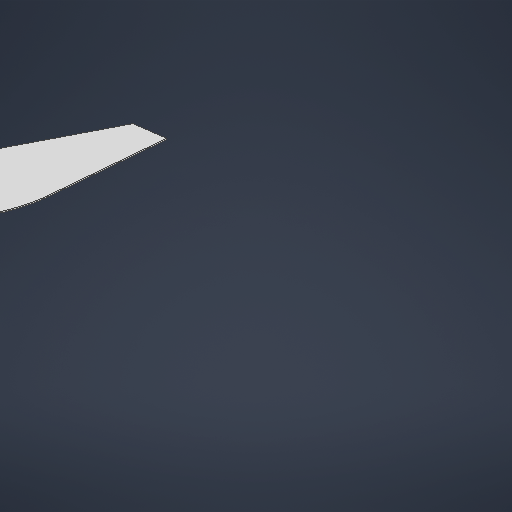
# Autodesk Inventor part: SLING
Saved by Autodesk Inventor 2026.2 (Build 302298010, 298A)
## iProperties
Created: 2026-04-04
Part Number: SLING
Material: Generic
Document SubType Name: Sheet Metal
Designer: 4aida
Density: 1 g/cm^3
Sheet Metal Rule: Default_mm
Appearance: Default
Author: 4aida
Autodesk Inventor part; units mm, degrees
ref_plane "YZ Plane" through (0, 0, 0) normal (1, 0, 0) x (0, 1, 0)
ref_plane "XZ Plane" through (0, 0, 0) normal (0, 1, 0) x (-1, 0, 0)
ref_plane "XY Plane" through (0, 0, 0) normal (0, 0, 1) x (1, 0, 0)
sketch "Sketch1" plane through (0, 0, 0) normal (0, 1, 0) x (-1, 0, 0)
  ellipse E0 centre (0, 0) end of major axis (0, -40) minor radius 25
  line L0 (23.4617, 13.8144) -> (8.75, 77.7778)
  line L1 (8.75, 77.7778) -> (-8.75, 77.7778)
  line L2 (-8.75, 77.7778) -> (-23.4617, 13.8144)
  line L3 (23.4617, -13.8144) -> (8.75, -77.7778)
  line L4 (8.75, -77.7778) -> (-8.75, -77.7778)
  line L5 (-8.75, -77.7778) -> (-23.4617, -13.8144)
  point P0 (0, 77.7778)
  point P1 (0, -77.7778)
  dimension "d0" = 25
  dimension "d1" = 40
  dimension "d2" = 77.7778
  dimension "d3" = 77.7778
  dimension "d5" = 17.5
  dimension "d7" = 17.5
  measures "d2" distance from line of point (0, 0) L1
  measures "d3" distance from line of L4 point (0, 0)
  measures "d5" distance of L0.end L1.end
  measures "d7" distance of L3.end L4.end
extrude "Plate1" add sketch "Sketch1" along normal blind 0.5
equation "\"d2\" = d3"
equation "\"d3\" = 3.11111 * d0"
equation "\"d5\" = d7"
equation "\"d8\" = Thickness"
equation "\"BendRadius\" = Thickness"
equation "\"BendReliefWidth\" = Thickness"
equation "\"BendReliefDepth\" = 0.5 * Thickness"
equation "\"CornerReliefSize\" = 4 * Thickness"
equation "\"MinimumRemnant\" = 2 * Thickness"
equation "\"TransitionRadius\" = BendRadius"
equation "\"JacobiRadiusSize\" = BendRadius"
equation "\"GapSize\" = Thickness"
equation "\"Thickness\" = 0.5"
body "Solid1"
